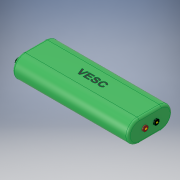
# Autodesk Inventor part: VESC
Saved by Autodesk Inventor 2019.2 (Build 232265000, 265)
## iProperties
Created: 2018-12-01
Part Number: VESC
Material: ABS Plastic
Document SubType Name: Modeling
Designer: Petar
Density: 1.06 g/cm^3
Appearance: Flaked Satin - Sea Green
Author: Petar
Autodesk Inventor part; units mm, degrees
ref_plane "YZ Plane" through (0, 0, 0) normal (1, 0, 0) x (0, 1, 0)
ref_plane "XZ Plane" through (0, 0, 0) normal (0, 1, 0) x (-1, 0, 0)
ref_plane "XY Plane" through (0, 0, 0) normal (0, 0, 1) x (1, 0, 0)
sketch "Sketch1" plane through (0, 0, 0) normal (0, 1, 0) x (-1, 0, 0)
  line L0 (133, -19.4873) -> (28, -19.4873)
  line L1 (28, -19.4873) -> (28, 20.5127)
  line L2 (28, 20.5127) -> (133, 20.5127)
  line L3 (133, 20.5127) -> (133, -19.4873)
  point P0 (0, 0)
  dimension "d0" = 105
  dimension "d1" = 40
  constraints: 8 end point, 2 parallel, 1 horizontal, 1 perpendicular
  measures "d0" distance of L1.end L2.end
  measures "d1" distance of L0.end L1.end
extrude "Extrusion1" add sketch "Sketch1" along normal blind 20
sketch "Sketch2" plane through (0, 20, 0) normal (0, 1, 0) x (1, 0, 0)
  line L0 (-133, 19.4873) -> (-133, -20.5127) projected
  line L1 (-28, -20.5127) -> (-28, 19.4873) projected
  line L2 (-130.5, 10.3911) -> (-30.5, 10.3911) construction
  line L3 (-30.5, 10.3911) -> (-30.5, -10.6646) construction
  line L4 (-30.5, -10.6646) -> (-130.5, -10.6646) construction
  line L5 (-130.5, -10.6646) -> (-130.5, 10.3911) construction
  line L6 (-90.6959, -3.1345) -> (-93.0465, 2.8655)
  line L7 (-93.0465, 2.8655) -> (-91.6014, 2.8655)
  line L8 (-91.6014, 2.8655) -> (-89.9322, -1.575)
  line L9 (-89.9322, -1.575) -> (-88.3178, 2.8655)
  line L10 (-88.3178, 2.8655) -> (-86.9047, 2.8655)
  line L11 (-86.9047, 2.8655) -> (-89.2645, -3.1345)
  line L12 (-89.2645, -3.1345) -> (-90.6959, -3.1345)
  line L13 (-86.2279, -3.1345) -> (-86.2279, 2.8655)
  line L14 (-86.2279, 2.8655) -> (-81.3438, 2.8655)
  line L15 (-81.3438, 2.8655) -> (-81.3438, 1.8503)
  line L16 (-81.3438, 1.8503) -> (-84.8971, 1.8503)
  line L17 (-84.8971, 1.8503) -> (-84.8971, 0.5195)
  line L18 (-84.8971, 0.5195) -> (-81.5907, 0.5195)
  line L19 (-81.5907, 0.5195) -> (-81.5907, -0.4957)
  line L20 (-81.5907, -0.4957) -> (-84.8971, -0.4957)
  line L21 (-84.8971, -0.4957) -> (-84.8971, -2.1192)
  line L22 (-84.8971, -2.1192) -> (-81.2157, -2.1192)
  line L23 (-81.2157, -2.1192) -> (-81.2157, -3.1345)
  line L24 (-81.2157, -3.1345) -> (-86.2279, -3.1345)
  line L25 (-80.42, -1.1772) -> (-79.1258, -1.0628)
  spline S0 degree 2 poles (-79.1258, -1.0628) (-79.0069, -1.6573) (-78.2934, -2.2153) (-77.6852, -2.2153) knots 0 0 0 1 2 2 2
  spline S1 degree 2 poles (-77.6852, -2.2153) (-77.045, -2.2153) (-76.391, -1.7214) (-76.391, -1.3875) knots 0 0 0 1 2 2 2
  spline S2 degree 2 poles (-76.391, -1.3875) (-76.391, -1.1726) (-76.6654, -0.8753) (-77.0084, -0.7656) knots 0 0 0 1 2 2 2
  spline S3 degree 2 poles (-77.0084, -0.7656) (-77.2416, -0.6924) (-78.0739, -0.5049) knots 0 0 0 1 1 1
  spline S4 degree 2 poles (-78.0739, -0.5049) (-79.1441, -0.2625) (-79.5739, 0.0896) knots 0 0 0 1 1 1
  spline S5 degree 2 poles (-79.5739, 0.0896) (-80.1822, 0.5835) (-80.1822, 1.2924) knots 0 0 0 1 1 1
  spline S6 degree 2 poles (-80.1822, 1.2924) (-80.1822, 1.7543) (-79.6105, 2.55) (-78.5358, 2.9661) (-77.7767, 2.9661) knots 0 0 0 1 2 3 3 3
  spline S7 degree 2 poles (-77.7767, 2.9661) (-76.5328, 2.9661) (-75.2797, 1.9783) (-75.2477, 1.1506) knots 0 0 0 1 2 2 2
  line L26 (-75.2477, 1.1506) -> (-76.5785, 1.0957)
  spline S8 degree 2 poles (-76.5785, 1.0957) (-76.6654, 1.5576) (-77.2279, 1.9646) (-77.7904, 1.9646) knots 0 0 0 1 2 2 2
  spline S9 degree 2 poles (-77.7904, 1.9646) (-78.3712, 1.9646) (-78.7005, 1.7497) knots 0 0 0 1 1 1
  spline S10 degree 2 poles (-78.7005, 1.7497) (-78.9108, 1.6079) (-78.9108, 1.3747) knots 0 0 0 1 1 1
  spline S11 degree 2 poles (-78.9108, 1.3747) (-78.9108, 1.1643) (-78.7142, 1.0088) knots 0 0 0 1 1 1
  spline S12 degree 2 poles (-78.7142, 1.0088) (-78.4627, 0.8168) (-76.5191, 0.4006) (-75.5861, -0.043) (-75.0602, -0.8159) (-75.0602, -1.3875) knots 0 0 0 1 2 3 4 4 4
  spline S13 degree 2 poles (-75.0602, -1.3875) (-75.0602, -1.8997) (-75.6913, -2.8006) (-76.8392, -3.2397) (-77.6989, -3.2397) knots 0 0 0 1 2 3 3 3
  spline S14 degree 2 poles (-77.6989, -3.2397) (-78.9474, -3.2397) (-80.2873, -2.1878) (-80.42, -1.1772) knots 0 0 0 1 2 2 2
  line L27 (-69.7188, -0.9256) -> (-68.4291, -1.2961)
  spline S15 degree 2 poles (-68.4291, -1.2961) (-68.7264, -2.2793) (-70.1075, -3.2351) (-71.1684, -3.2351) knots 0 0 0 1 2 2 2
  spline S16 degree 2 poles (-71.1684, -3.2351) (-72.4809, -3.2351) (-74.173, -1.6025) (-74.173, -0.1893) knots 0 0 0 1 2 2 2
  spline S17 degree 2 poles (-74.173, -0.1893) (-74.173, 1.3107) (-72.4718, 2.9661) (-71.0861, 2.9661) knots 0 0 0 1 2 2 2
  spline S18 degree 2 poles (-71.0861, 2.9661) (-69.8788, 2.9661) (-69.1242, 2.3168) knots 0 0 0 1 1 1
  spline S19 degree 2 poles (-69.1242, 2.3168) (-68.6715, 1.9326) (-68.4474, 1.2146) knots 0 0 0 1 1 1
  line L28 (-68.4474, 1.2146) -> (-69.7645, 0.9265)
  spline S20 degree 2 poles (-69.7645, 0.9265) (-69.8834, 1.393) (-70.6242, 1.9326) (-71.1547, 1.9326) knots 0 0 0 1 2 2 2
  spline S21 degree 2 poles (-71.1547, 1.9326) (-71.8864, 1.9326) (-72.8011, 0.9768) (-72.8011, -0.0979) knots 0 0 0 1 2 2 2
  spline S22 degree 2 poles (-72.8011, -0.0979) (-72.8011, -1.2366) (-71.9002, -2.2015) (-71.1822, -2.2015) knots 0 0 0 1 2 2 2
  spline S23 degree 2 poles (-71.1822, -2.2015) (-70.6517, -2.2015) (-69.8834, -1.5842) (-69.7188, -0.9256) knots 0 0 0 1 2 2 2
  point P0 (0, 0)
  dimension "d4" = 2.5
  dimension "d5" = 2.5
  constraints: 2 other
  measures "d4" distance between parallel lines of L1 L3
  measures "d5" distance between parallel lines of L0 L5
emboss "Emboss1" sketch "Sketch2" operation cut depth 0.1 direction (0, -1, 0)
sketch "Sketch3" plane through (-133, 0, -19.4873) normal (-1, 0, 0) x (0, 0, 1)
  line L0 (40, 0) -> (0, 0) projected
  line L1 (40, 0) -> (40, 20) projected
  line L2 (0, 20) -> (40, 20) projected
  line L3 (0, 0) -> (0, 20) projected
  line L4 (20, 20) -> (20, 0) construction
  circle A0 centre (10, 10) radius 2.5
  line L5 (0, 10) -> (40, 10) construction
  circle A1 centre (30, 10) radius 2.5
  circle A2 centre (20, 10) radius 2.5
  point P0 (19.4873, 0)
  dimension "d8" = 5
  dimension "d9" = 10
  dimension "d10" = 5
  constraints: 5 midpoint, 4 end point, 3 centre point, 1 point on line, 1 symmetric about line, 1 other
  measures "d8" diameter of A0
  measures "d9" distance from line of A0.centre L3
  measures "d10" diameter of A2
extrude "Extrusion2" add sketch "Sketch3" along normal blind 5 contours A0 | A1 | A2
sketch "Sketch4" plane through (-28, 0, 20.5127) normal (1, 0, 0) x (0, 0, -1)
  line L0 (40, 0) -> (40, 20) projected
  line L1 (0, 20) -> (40, 20) projected
  line L2 (0, 0) -> (0, 20) projected
  line L3 (0, 10) -> (40, 10) construction
  line L4 (20, 20) -> (20, 0) construction
  line L5 (0, 0) -> (40, 0) projected
  circle A0 centre (15, 10) radius 2.5
  circle A1 centre (25, 10) radius 2.5
  point P0 (20.5127, 0)
  dimension "d13" = 5
  dimension "d14" = 5
  dimension "d15" = 15
  dimension "d16" = 15
  constraints: 4 end point, 4 midpoint, 2 centre point, 2 point on line
  measures "d13" diameter of A0
  measures "d14" diameter of A1
  measures "d15" distance from line of L2 A0.centre
  measures "d16" distance from line of L0 A1.centre
extrude "Extrusion3" add sketch "Sketch4" along normal blind 1 contours A0 | A1
fillet "Fillet1" radius 10 4 edges at (-80.5, 20, 20.5127) (-80.5, 0, 20.5127) (-80.5, 20, -19.4873) (-80.5, 0, -19.4873)
fillet "Fillet2" radius 2 16 edges at (-28, 10, -19.4873) (-28, 2.9289, -16.5583) (-28, 17.0711, -16.5583) (-28, 0, 0.5127) (-28, 2.9289, 17.5838) (-28, 17.0711, 17.5838) (-28, 10, 20.5127) (-28, 20, 0.5127) (-133, 10, 20.5127) (-133, 2.9289, 17.5838) (-133, 17.0711, 17.5838) (-133, 0, 0.5127) (-133, 10, -19.4873) (-133, 2.9289, -16.5583) (-133, 17.0711, -16.5583) (-133, 20, 0.5127)
chamfer "Chamfer1" distance 0.1 angle 45 47 edges at (-88.0846, 20, 0.1345) (-89.125, 20, -0.6453) (-90.7668, 20, -0.6453) (-92.3239, 20, -2.8655) (-91.8712, 20, 0.1345) (-89.9802, 20, 3.1345) (-87.6113, 20, -2.8655) (-83.7858, 20, -2.8655) (-86.2279, 20, 0.1345) (-83.2439, 20, -0.5195) (-80.0242, 20, -0.6258) (-79.4498, 20, -2.5696) (-76.0403, 20, -2.5677) (-76.9624, 20, -1.7722) (-78.2863, 20, -1.9159) (-78.8578, 20, -1.5858) (-78.8609, 20, -1.1766) (-76.2703, 20, -0.2712) (-75.8666, 20, 2.8201) (-79.5413, 20, 2.7705) (-76.7733, 20, 2.0069) (-76.5371, 20, 1.0146) (-78.6488, 20, 1.9374) (-79.7729, 20, 1.12) (-81.5907, 20, -0.0119) (-83.2439, 20, 0.4957) (-81.3438, 20, -2.3579) (-84.8971, 20, 1.3075) (-83.0564, 20, 2.1192) (-83.7218, 20, 3.1345) (-81.2157, 20, 2.6268) (-75.9131, 20, -1.1232) (-72.4407, 20, 1.6098) (-70.2382, 20, 1.8685) (-72.4173, 20, -1.3703) (-70.2639, 20, -1.6701) (-73.3529, 20, 2.3934) (-73.3532, 20, -2.1079) (-70.0344, 20, -2.8175) (-69.4312, 20, 2.767) (-69.1059, 20, -1.0706) (-69.0739, 20, 1.1108) (-83.1204, 20, -1.8503) (-84.8971, 20, -1.1849) (-78.8914, 20, 0.2705) (-77.4721, 20, 0.6442) (-68.7154, 20, -1.8274)
sketch "Sketch5" plane through (-27, 10, -4.4873) normal (1, 0, 0) x (0, 0, -1)
  circle A0 centre (0, 0) radius 2.5 projected
sketch "Sketch6" plane through (-27, 10, 5.5127) normal (1, 0, 0) x (0, 0, -1)
  circle A0 centre (0, 0) radius 2.5 projected
sketch "Sketch7" plane through (-138, 10, 10.5127) normal (-1, 0, 0) x (0, 0, 1)
  circle A0 centre (0, 0) radius 2.5 projected
sketch "Sketch8" plane through (-138, 10, 0.5127) normal (-1, 0, 0) x (0, 0, 1)
  circle A0 centre (0, 0) radius 2.5 projected
sketch "Sketch9" plane through (-138, 10, -9.4873) normal (-1, 0, 0) x (0, 0, 1)
  circle A0 centre (0, 0) radius 2.5 projected
body "Solid1"
